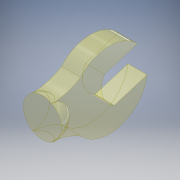
# Autodesk Inventor part: Spanner
Saved by Autodesk Inventor 2017 (Build 210142000, 142)
## iProperties
Created: 2021-02-25
Part Number: Spanner
Material: Generic
Document SubType Name: Modeling
Designer: Lenovo Y900
Density: 1 g/cm^3
Appearance: Clear - Yellow
Author: Lenovo Y900
Autodesk Inventor part; units mm, degrees
ref_plane "YZ Plane" through (0, 0, 0) normal (1, 0, 0) x (0, 1, 0)
ref_plane "XZ Plane" through (0, 0, 0) normal (0, 1, 0) x (-1, 0, 0)
ref_plane "XY Plane" through (0, 0, 0) normal (0, 0, 1) x (1, 0, 0)
sketch "Sketch1" plane through (0, 0, 0) normal (0, 0, 1) x (1, 0, 0)
  arc A0 (7.5, 0) -> (-7.5, 0) centre (0, 0) ccw
  line L0 (-7.5, 0) -> (7.5, 0)
  dimension "d2" = 7.5
  constraints: 2 end point, 2 point on circle, 1 centre point, 1 coincident, 1 horizontal
  measures "d2" distance of L0.start point (0, 0)
revolve "Revolution1" add sketch "Sketch1" angle 180 mid plane about axis through (-7.5, 0, 0) along (1, 0, 0)
sketch "Sketch2" plane through (0, 0, 0) normal (1, 0, 0) x (0, 1, 0)
  line L0 (24.4009, -6.216) -> (37.3287, -2.2636)
  line L1 (33.5279, 10.1684) -> (20.6001, 6.216)
  arc A0 (20.6001, 6.216) -> (24.4009, -6.216) centre (28.4534, 1.82) ccw
  arc A1 (33.5279, 10.1684) -> (11.2086, 9.8739) centre (22.5005, 0) ccw
  arc A2 (11.6815, -10.3899) -> (37.3287, -2.2636) centre (22.5005, 0) ccw
  arc A3 (11.6815, -10.3899) -> (0, -6.4952) centre (-1.1685, -29.4655) ccw
  arc A4 (0, 6.4952) -> (11.2086, 9.8739) centre (-0.8152, 29.4807) ccw
  line L2 (0, -6.4952) -> (0, 6.4952)
  line L3 (0, 7.5) -> (0, -7.5) projected
  point P0 (0, 0)
  dimension "d15" = 23
  dimension "d16" = 23
  constraints: 10 point on circle, 6 end point, 5 centre point, 1 collinear, 1 parallel
  measures "d15" radius of A3
  measures "d16" radius of A4
extrude "Extrusion1" add sketch "Sketch2" along normal mid plane 7.5
body "Solid1"
